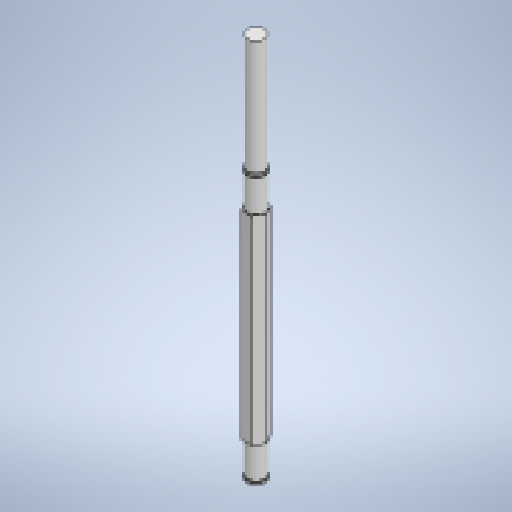
# Autodesk Inventor part: NVPH-201 shredder shaft
Saved by Autodesk Inventor 2025.1 (Build 291241020, 241B)
## iProperties
Created: 2024-12-04
Part Number: NVPH-201 shredder shaft
Material: Generic
Document SubType Name: Modeling
Designer: DELL
Density: 1 g/cm^3
Appearance: Default
Author: DELL
Autodesk Inventor part; units mm, degrees
ref_plane "YZ Plane" through (0, 0, 0) normal (1, 0, 0) x (0, 1, 0)
ref_plane "XZ Plane" through (0, 0, 0) normal (0, 1, 0) x (-1, 0, 0)
ref_plane "XY Plane" through (0, 0, 0) normal (0, 0, 1) x (1, 0, 0)
sketch "Sketch1" plane through (0, 0, 0) normal (0, 0, 1) x (1, 0, 0)
  line L0 (-9.2376, -16) -> (-18.4752, 0)
  line L1 (-18.4752, 0) -> (-9.2376, 16)
  line L2 (-9.2376, 16) -> (9.2376, 16)
  line L3 (9.2376, 16) -> (18.4752, 0)
  line L4 (18.4752, 0) -> (9.2376, -16)
  line L5 (9.2376, -16) -> (-9.2376, -16)
  point P0 (0, 0)
  point P1 (0, 0)
  dimension "d0" = 32
  constraints: 12 end point, 1 coincident, 1 horizontal, 13 other
  measures "d0" distance between parallel lines of L5 L2
extrude "Extrusion1" add sketch "Sketch1" along normal mid plane 334
sketch "Sketch3" plane through (0, 0, 0) normal (0, 1, 0) x (-1, 0, 0)
  line L0 (0, -227) -> (0, 0)
  line L1 (0, 0) -> (0, 420)
  line L2 (0, 420) -> (-14, 420)
  line L3 (-14, 420) -> (-14, 227)
  line L4 (-14, 227) -> (-15, 227)
  line L5 (-15, 227) -> (-15, 0)
  line L6 (-15, 0) -> (-15, -227)
  line L7 (-15, -227) -> (0, -227)
  line L8 (-15, -223) -> (-14, -223)
  line L9 (-14, -223) -> (-14, -221)
  line L10 (-14, -221) -> (-15, -221)
  line L11 (-15, -221) -> (-15, -223)
  line L12 (-14, 416) -> (-13, 416)
  line L13 (-13, 416) -> (-13, 414)
  line L14 (-13, 414) -> (-14, 414)
  line L15 (-14, 414) -> (-14, 416)
  line L16 (-15, 223) -> (-14, 223)
  line L17 (-14, 223) -> (-14, 221)
  line L18 (-14, 221) -> (-15, 221)
  line L19 (-15, 221) -> (-15, 223)
  point P0 (-15, 221)
  dimension "d8" = 30
  dimension "d9" = 227
  dimension "d10" = 420
  dimension "d12" = 28
  dimension "d14" = 4
  dimension "d15" = 2
  dimension "d16" = 26
  dimension "d17" = 2
  dimension "d18" = 4
  dimension "d19" = 28
  dimension "d20" = 227
  dimension "d21" = 2
  dimension "d22" = 4
  dimension "d23" = 28
  constraints: 40 end point, 8 perpendicular, 6 parallel, 5 point on line, 3 horizontal, 1 vertical
  measures "d8" diameter of L6 L0
  measures "d9" distance from line of L0.end L7
  measures "d10" distance of L1.end L0.end
  measures "d12" diameter of L3 L1
  measures "d14" distance between parallel lines of L2 L12
  measures "d15" distance of L12.end L13.end
  measures "d16" diameter of L13 L1
  measures "d17" distance of L8.end L9.end
  measures "d18" distance between parallel lines of L7 L8
  measures "d19" diameter of L9 L0
  measures "d20" distance from line of L0.end L4
  measures "d21" distance of L16.end L17.end
  measures "d22" distance between parallel lines of L4 L16
  measures "d23" diameter of L17 L1
revolve "Revolution1" add sketch "Sketch3" angle 360 about axis through (0, 0, -227) along (0, 0, 1) contours L7 L6 L8 L9 L10 L5 L18 L17 L16 L4 L3 L14 L13 L12 L2 L1 L0 | L12 L13 L14 L3
equation "\"d23\" = d19"
body "Solid1"
